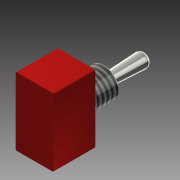
# Autodesk Inventor part: switch
Saved by Autodesk Inventor 2015 (Build 190159000, 159)
## iProperties
Created: 2015-10-31
Part Number: switch
Material: Generic
Document SubType Name: Modeling
Designer: James
Density: 1 g/cm^3
Appearance: Default
Author: James
Autodesk Inventor part; units mm, degrees
ref_plane "YZ Plane" through (0, 0, 0) normal (1, 0, 0) x (0, 1, 0)
ref_plane "XZ Plane" through (0, 0, 0) normal (0, 1, 0) x (-1, 0, 0)
sketch "Sketch1" plane through (0, 0, 0) normal (0, 1, 0) x (-1, 0, 0)
  line L0 (8, -14.25) -> (8, 14.25)
  line L1 (8, 14.25) -> (-8, 14.25)
  line L2 (-8, 14.25) -> (-8, -14.25)
  line L3 (-8, -14.25) -> (8, -14.25)
  line L4 (8, -14.25) -> (-8, 14.25) construction
  line L5 (8, 14.25) -> (-8, -14.25) construction
  point P0 (0, 0)
  dimension "d0" = 28.5
  dimension "d1" = 16
  constraints: 12 end point, 2 midpoint, 2 parallel, 1 perpendicular, 1 vertical
  measures "d0" distance of L0.start L0.end
  measures "d1" distance of L1.end L0.end
extrude "Extrusion1" add sketch "Sketch1" along normal blind 17.4
fillet "Fillet1" radius 0.5 4 edges at (-8, 8.7, 14.25) (8, 8.7, 14.25) (8, 8.7, -14.25) (-8, 8.7, -14.25)
sketch "Sketch2" plane through (0, 17.4, 0) normal (0, 1, 0) x (1, 0, 0)
  circle A0 centre (0, 0) radius 6.25
  dimension "d5" = 12.5
  constraints: 1 centre point, 1 coincident
  measures "d5" diameter of A0
extrude "Extrusion2" add sketch "Sketch2" along normal blind 12
sketch "Sketch3" plane through (0, 29.4, 0) normal (0, 1, 0) x (1, 0, 0)
  circle A0 centre (0, 0) radius 2.25
  dimension "d8" = 4.5
  constraints: 1 centre point, 1 coincident
  measures "d8" diameter of A0
ref_plane "Work Plane1" through (0, 46.4, 0) normal (0, 1, 0) x (1, 0, 0)
sketch "Sketch4" plane through (0, 46.4, 0) normal (0, 1, 0) x (1, 0, 0)
  circle A0 centre (0, 0) radius 3.05
  dimension "d10" = 6.1
  constraints: 1 centre point, 1 coincident
  measures "d10" diameter of A0
loft "Loft1" add profiles "Sketch3", "Sketch4"
fillet "Fillet2" radius 2 1 edges at (-3.05, 46.4, 0)
chamfer "Chamfer1" distance 0.5 angle 45 1 edges at (-6.25, 29.4, 0)
thread "Thread2" size "M14x2" class "6g" standard "ANSI Metric M Profile" full length
body "Solid1"
